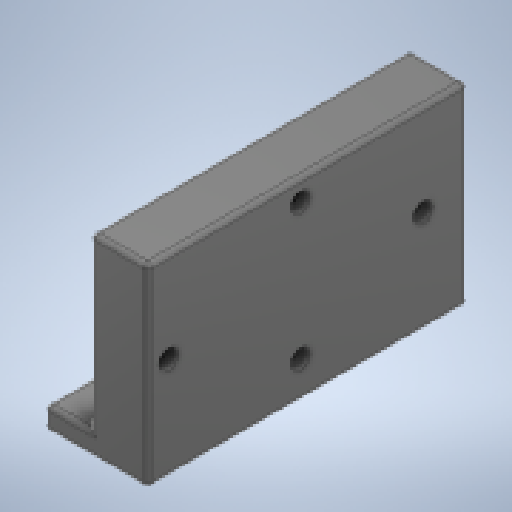
# Autodesk Inventor part: gripper_bracket
Saved by Autodesk Inventor 2026.2 (Build 302298010, 298A)
## iProperties
Created: 2026-04-13
Part Number: gripper_bracket
Material: ABS Plastic
Document SubType Name: Modeling
Designer: chris
Density: 1.06 g/cm^3
Appearance: Smooth - White
Author: chris
Autodesk Inventor part; units mm, degrees
ref_plane "YZ Plane" through (0, 0, 0) normal (1, 0, 0) x (0, 1, 0)
ref_plane "XZ Plane" through (0, 0, 0) normal (0, 1, 0) x (-1, 0, 0)
ref_plane "XY Plane" through (0, 0, 0) normal (0, 0, 1) x (1, 0, 0)
sketch "Sketch1" plane through (0, 0, 0) normal (0, 1, 0) x (-1, 0, 0)
  line L0 (15, 43) -> (-15, 43)
  line L1 (-15, 43) -> (-15, -43)
  line L2 (-15, -43) -> (15, -43)
  line L3 (15, -43) -> (15, 43)
  line L4 (15, 43) -> (-15, -43) construction
  line L5 (-15, 43) -> (15, -43) construction
  point P0 (0, 0)
  dimension "d0" = 30
  dimension "d1" = 86
  constraints: 12 end point, 2 midpoint, 2 parallel, 1 horizontal, 1 perpendicular
  measures "d0" distance of L2.end L1.end
  measures "d1" distance of L1.end L0.end
extrude "Extrusion1" add sketch "Sketch1" along normal blind 10
sketch "Sketch5" plane through (0, 10, 0) normal (0, 1, 0) x (1, 0, 0)
  line L0 (-15, 65) -> (-15, 43)
  line L1 (-15, 43) -> (15, 43)
  line L2 (15, 43) -> (15, -43)
  line L3 (15, -43) -> (-15, -43)
  line L4 (-15, -43) -> (-15, -65)
  line L5 (-15, -65) -> (25, -65)
  line L6 (25, -65) -> (25, 65)
  line L7 (25, 65) -> (-15, 65)
  line L8 (-15, 43) -> (-15, -43) projected
  line L9 (-15, -43) -> (15, -43) projected
  line L10 (15, 43) -> (-15, 43) projected
  line L11 (15, -43) -> (15, 43) projected
  point P0 (0, 0)
  dimension "d22" = 130
  dimension "d23" = 40
  dimension "d24" = 22
  constraints: 16 end point, 7 perpendicular, 5 collinear, 1 vertical
  measures "d22" distance of L5.end L6.end
  measures "d23" distance of L4.end L5.end
  measures "d24" distance between parallel lines of L5 L3
extrude "Extrusion5" add sketch "Sketch5" against normal blind 10 contours L7 L6 L5 L4 L3 L2 L1 L0
sketch "Sketch6" plane through (25, 10, 65) normal (1, 0, 0) x (0, 0, -1)
  line L0 (130, 75) -> (0, 75)
  line L1 (0, 75) -> (0, 0)
  line L2 (0, 0) -> (130, 0)
  line L3 (130, 0) -> (130, 75)
  line L4 (0, 0) -> (130, 0) projected
  line L5 (130, 0) -> (130, -10) projected
  line L6 (0, 0) -> (0, -10) projected
  point P0 (65, -10)
  dimension "d27" = 75
  constraints: 8 end point, 3 collinear, 2 parallel, 1 horizontal, 1 perpendicular
  measures "d27" distance of L0.end L1.end
extrude "Extrusion6" add sketch "Sketch6" against normal blind 10
sketch "Sketch7" plane through (15, 10, 65) normal (-1, 0, 0) x (0, 0, 1)
  line L0 (-127, 0) -> (-3, 0)
  line L1 (-3, 0) -> (-3, 72)
  line L2 (-3, 72) -> (-127, 72)
  line L3 (-127, 72) -> (-127, 0)
  line L4 (-130, 0) -> (0, 0)
  line L5 (0, 0) -> (0, 75)
  line L6 (0, 75) -> (-130, 75)
  line L7 (-130, 75) -> (-130, 0)
  line L8 (-130, 0) -> (0, 0) projected
  line L9 (-130, 75) -> (-130, 0) projected
  line L10 (0, 0) -> (0, 75) projected
  line L11 (0, 75) -> (-130, 75) projected
  point P0 (-65, -10)
  point P1 (-3, 0)
  dimension "d30" = 3
  dimension "d31" = 3
  dimension "d32" = 3
  constraints: 16 end point, 5 collinear, 4 parallel, 2 horizontal, 2 perpendicular
  measures "d30" distance between parallel lines of L6 L2
  measures "d31" distance between parallel lines of L5 L1
  measures "d32" distance between parallel lines of L7 L3
extrude "Extrusion7" add sketch "Sketch7" along normal blind 15 contours L4 L7 L6 L5 L1 L2 L3
sketch "Sketch8" plane through (15, 10, 65) normal (-1, 0, 0) x (0, 0, 1)
  circle A0 centre (-120.75, 35) radius 4.25
  line L0 (-127, 0) -> (-127, 72) projected
  line L1 (-130, 0) -> (0, 0) projected
  circle A1 centre (-67, 6.25) radius 4.25
  circle A2 centre (-67, 65.75) radius 4.25
  circle A3 centre (-9.25, 35) radius 4.25
  line L2 (-3, 72) -> (-3, 0) projected
  line L3 (-127, 72) -> (-3, 72) projected
  point P0 (-65, -10)
  dimension "d35" = 8.5
  dimension "d36" = 6.25
  dimension "d37" = 35
  dimension "d38" = 8.5
  dimension "d39" = 8.5
  dimension "d40" = 8.5
  dimension "d41" = 6.25
  dimension "d42" = 6.25
  dimension "d43" = 6.25
  dimension "d44" = 60
  dimension "d45" = 60
  dimension "d46" = 35
  constraints: 4 centre point
  measures "d35" diameter of A0
  measures "d36" distance from line of L0 A0.centre
  measures "d37" distance from line of L1 A0.centre
  measures "d38" diameter of A1
  measures "d39" diameter of A2
  measures "d40" diameter of A3
  measures "d41" distance from line of L2 A3.centre
  measures "d42" distance from line of L3 A2.centre
  measures "d43" distance from line of L1 A1.centre
  measures "d44" distance from line of L0 A1.centre
  measures "d45" distance from line of L0 A2.centre
  measures "d46" distance from line of L1 A3.centre
extrude "Extrusion8" cut sketch "Sketch8" against normal blind 10 contours A0 | A1 | A2 | A3
sketch "Sketch9" plane through (-15, 10, -65) normal (-1, 0, 0) x (0, 0, 1)
  line L0 (130, -10) -> (0, -10) projected
  line L1 (130, 0) -> (130, -10) projected
  line L2 (0, 0) -> (130, 0) projected
  line L3 (0, 0) -> (0, -10) projected
  point P0 (65, -10)
extrude "Extrusion9" add sketch "Sketch9" along normal blind 5
sketch "Sketch10" plane through (0, 0, 0) normal (0, -1, 0) x (1, 0, 0)
  circle A0 centre (-10, -7.5) radius 2.05
  circle A1 centre (5, 7.5) radius 2.05
  circle A2 centre (-10, 7.5) radius 2.05
  circle A3 centre (5, -7.5) radius 2.05
  line L0 (-20, -65) -> (-20, 65) projected
  point P0 (0, 0)
  dimension "d51" = 4.1
  dimension "d52" = 4.1
  dimension "d53" = 4.1
  dimension "d54" = 4.1
  dimension "d55" = 10
  dimension "d56" = 25
  dimension "d57" = 25
  dimension "d58" = 10
  dimension "d59" = 7.5
  dimension "d60" = 7.5
  dimension "d61" = 7.5
  dimension "d62" = 7.5
  constraints: 4 centre point
  measures "d51" diameter of A0
  measures "d52" diameter of A1
  measures "d53" diameter of A2
  measures "d54" diameter of A3
  measures "d55" distance from line of L0 A0.centre
  measures "d56" distance from line of L0 A3.centre
  measures "d57" distance from line of L0 A1.centre
  measures "d58" distance from line of L0 A2.centre
  measures "d59" vertical distance of A0.centre point (0, 0)
  measures "d60" vertical distance of point (0, 0) A2.centre
  measures "d61" vertical distance of point (0, 0) A1.centre
  measures "d62" vertical distance of point (0, 0) A3.centre
extrude "Extrusion10" cut sketch "Sketch10" against normal blind 10
sketch "Sketch11" plane through (0, 10, 0) normal (0, 1, 0) x (1, 0, 0)
  circle A0 centre (5, 7.5) radius 2.05 projected
  circle A1 centre (5, -7.5) radius 2.05 projected
  circle A2 centre (-10, 7.5) radius 2.05 projected
  circle A3 centre (-10, -7.5) radius 2.05 projected
  circle A4 centre (-10, 7.5) radius 5
  circle A5 centre (5, 7.5) radius 5
  circle A6 centre (-10, -7.5) radius 5
  circle A7 centre (5, -7.5) radius 5
  point P0 (0, 0)
  dimension "d65" = 10
  dimension "d66" = 10
  dimension "d67" = 10
  dimension "d68" = 10
  constraints: 4 centre point, 4 coincident
  measures "d65" diameter of A4
  measures "d66" diameter of A5
  measures "d67" diameter of A6
  measures "d68" diameter of A7
extrude "Extrusion11" cut sketch "Sketch11" against normal blind 5
sketch "Sketch12" plane through (15, 82, -62) normal (-1, 0, 0) x (0, 0, 1)
  circle A0 centre (117.75, -37) radius 4.25 projected
  circle A1 centre (60, -6.25) radius 4.25 projected
  circle A2 centre (60, -65.75) radius 4.25 projected
  circle A3 centre (6.25, -37) radius 4.25 projected
  circle A4 centre (117.75, -37) radius 6.25
  circle A5 centre (60, -6.25) radius 6.25
  circle A6 centre (6.25, -37) radius 6.25
  circle A7 centre (60, -65.75) radius 6.25
  point P0 (62, -82)
  point P1 (64.25, -65.75)
  dimension "d73" = 12.5
  dimension "d74" = 12.5
  dimension "d75" = 12.5
  dimension "d76" = 12.5
  constraints: 4 centre point, 4 coincident, 1 horizontal alignment
  measures "d73" diameter of A4
  measures "d74" diameter of A5
  measures "d75" diameter of A6
  measures "d76" diameter of A7
extrude "Extrusion12" cut sketch "Sketch12" against normal blind 5
sketch "Sketch16" plane through (25, 0, -65) normal (0, 0, -1) x (-1, 0, 0)
  line L0 (0, 85) -> (25, 85)
  line L1 (25, 85) -> (25, 0)
  line L2 (25, 0) -> (0, 0)
  line L3 (0, 0) -> (0, 85)
  line L4 (0, 85) -> (25, 85) projected
  line L5 (0, 0) -> (45, 0) projected
  line L6 (25, 85) -> (25, 10) projected
  line L7 (0, 0) -> (0, 85) projected
  point P0 (25, 0)
  constraints: 8 end point, 4 collinear, 2 parallel, 1 horizontal, 1 perpendicular
extrude "Extrusion16" add sketch "Sketch16" along normal blind 10
sketch "Sketch17" plane through (25, 0, -75) normal (0, 0, -1) x (-1, 0, 0)
  circle A0 centre (21, 65) radius 1.55
  circle A1 centre (21, 35) radius 1.55
  line L0 (25, 0) -> (25, 85) projected
  line L1 (25, 85) -> (0, 85) projected
  circle A2 centre (21, 50) radius 1.55
  dimension "d95" = 3.1
  dimension "d96" = 3.1
  dimension "d97" = 4
  dimension "d98" = 4
  dimension "d99" = 20
  dimension "d100" = 30
  dimension "d107" = 3.1
  dimension "d108" = 4
  dimension "d109" = 35
  constraints: 3 centre point
  measures "d95" diameter of A0
  measures "d96" diameter of A1
  measures "d97" distance from line of L0 A0.centre
  measures "d98" distance from line of L0 A1.centre
  measures "d99" distance from line of A0.centre L1
  measures "d100" distance of A1.centre A0.centre
  measures "d107" diameter of A2
  measures "d108" distance from line of L0 A2.centre
  measures "d109" distance from line of L1 A2.centre
extrude "Extrusion17" cut sketch "Sketch17" against normal blind 13
sketch "Sketch18" plane through (0, 82, -62) normal (0, 0, 1) x (1, 0, 0)
  circle A0 centre (4, -17) radius 1.55 projected
  circle A1 centre (4, -47) radius 1.55 projected
  circle A2 centre (4, -17) radius 3.5
  circle A3 centre (4, -47) radius 3.5
  circle A4 centre (4, -32) radius 1.55 projected
  circle A5 centre (4, -32) radius 3.5
  point P0 (0, -82)
  dimension "d103" = 7
  dimension "d104" = 7
  dimension "d110" = 7
  constraints: 3 centre point, 3 coincident
  measures "d103" diameter of A2
  measures "d104" diameter of A3
  measures "d110" diameter of A5
extrude "Extrusion18" cut sketch "Sketch18" against normal blind 5 contours A0 | A1 | A2 | A3 | A5
fillet "Fillet3" radius 2 20 edges at (2.5, 0, 65) (-20, 5, 65) (-10, 10, 65) (0, 47.5, 65) (12.5, 85, 65) (25, 42.5, 65) (25, 85, -5) (0, 85, -5) (25, 42.5, -75) (0, 42.5, -75) (12.5, 85, -75) (12.5, 0, -75) (25, 0, -5) (-20, 10, 0) (-20, 0, 0) (-20, 5, -65) (0, 5, -65) (-10, 0, -65) (0, 0, -70) (-10, 10, -65)
body "Solid1"
